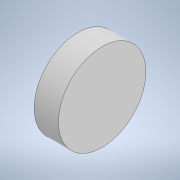
# Autodesk Inventor part: 큰 원통
Saved by Autodesk Inventor 2022 (Build 260153000, 153)
## iProperties
Created: 2022-10-28
Part Number: 큰 원통
Material: 일반
Document SubType Name: Modeling
Designer: gogin
Density: 1 g/cm^3
Appearance: 기본값
Author: gogin
Autodesk Inventor part; units mm, degrees
ref_plane "YZ Plane" through (0, 0, 0) normal (1, 0, 0) x (0, 1, 0)
ref_plane "XZ Plane" through (0, 0, 0) normal (0, 1, 0) x (-1, 0, 0)
ref_plane "XY Plane" through (0, 0, 0) normal (0, 0, 1) x (1, 0, 0)
sketch "스케치3" plane through (0, 0, 0) normal (1, 0, 0) x (0, 1, 0)
  circle A0 centre (0, 0) radius 4.5
  dimension "d0" = 9
  dimension "d1" = 0
  dimension "d2" = 0
  constraints: 1 centre point
  measures "d0" diameter of A0
  measures "d1" distance of point (0, 0) A0.centre
  measures "d2" distance of point (0, 0) A0.centre
extrude "돌출1" add sketch "스케치3" along normal blind 2.5
